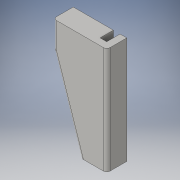
# Autodesk Inventor part: Right Leg, Front part
Saved by Autodesk Inventor 2016 (Build 200138000, 138)
## iProperties
Created: 2017-11-04
Part Number: Right Leg, Front part
Material: Generic
Document SubType Name: Modeling
Designer: mathaetaes
Density: 1 g/cm^3
Appearance: Default
Author: mathaetaes
Autodesk Inventor part; units mm, degrees
ref_plane "YZ Plane" through (0, 0, 0) normal (1, 0, 0) x (0, 1, 0)
ref_plane "XZ Plane" through (0, 0, 0) normal (0, 1, 0) x (-1, 0, 0)
ref_plane "XY Plane" through (0, 0, 0) normal (0, 0, 1) x (1, 0, 0)
sketch "Sketch1" plane through (0, 0, 0) normal (0, 0, 1) x (1, 0, 0)
  line L0 (-51.3998, 21.3475) -> (-0.5998, 21.3475)
  line L1 (-0.5998, 21.3475) -> (-0.5998, -80.2525)
  line L2 (-0.5998, -80.2525) -> (-25.9998, -80.2525)
  line L3 (-25.9998, -80.2525) -> (-51.3998, -4.0525)
  line L4 (-51.3998, -4.0525) -> (-51.3998, 21.3475)
  dimension "d1" = 50.8
  dimension "d3" = 25.4
  dimension "d4" = 76.2
  dimension "d5" = 25.4
  constraints: 10 end point, 2 perpendicular, 1 horizontal, 1 parallel
  measures "d1" distance of L0.start L0.end
  measures "d3" distance of L1.end L2.end
  measures "d4" distance from line of L2 L3.end
  measures "d5" distance of L3.end L0.start
extrude "Extrusion1" add sketch "Sketch1" along normal blind 19.05
sketch "Sketch2" plane through (-51.3998, 21.3475, 0) normal (0, 1, 0) x (1, 0, 0)
  line L0 (0, 0) -> (50.8, 0) projected
  line L1 (38.1, 0) -> (44.45, 0)
  line L2 (44.45, 0) -> (44.45, -12.7)
  line L3 (44.45, -12.7) -> (38.1, -12.7)
  line L4 (38.1, -12.7) -> (38.1, 0)
  line L5 (50.8, 0) -> (50.8, -19.05) projected
  point P0 (51.3998, 0)
  dimension "d8" = 6.35
  dimension "d10" = 6.35
  dimension "d11" = 12.7
  constraints: 8 end point, 2 parallel, 1 horizontal, 1 perpendicular, 1 point on line
  measures "d8" distance between parallel lines of L5 L2
  measures "d10" distance of L2.end L3.end
  measures "d11" distance of L1.end L2.end
extrude "Extrusion2" cut sketch "Sketch2" against normal blind 101.6
fillet "Fillet1" radius 3.175 3 edges at (-0.5998, -29.4525, 19.05) (-38.6998, -42.1525, 19.05) (-51.3998, 8.6475, 19.05)
equation "\"d12\" = d5 + d4"
body "Solid1"
